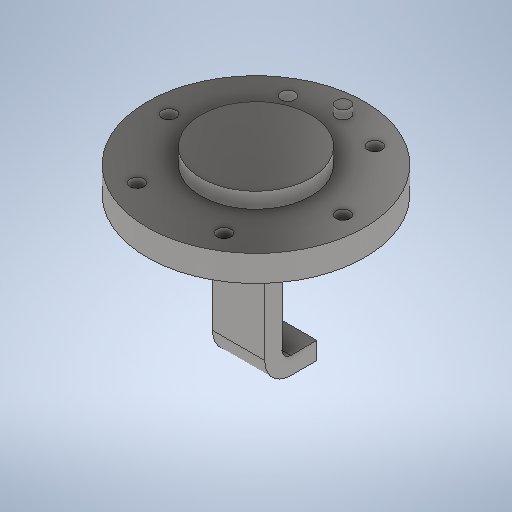
# Autodesk Inventor part: EndEffector
Saved by Autodesk Inventor 2025.1 (Build 291241000, 241)
## iProperties
Created: 2025-01-29
Part Number: EndEffector
Material: Steel, High Strength, Low Alloy
Document SubType Name: Modeling
Designer: yovan
Mass: 2366.38 g
Surface Area: 474.303 cm^2
Volume: 301.45 cm^3
Density: 7.85 g/cm^3
Appearance: Steel - Polished
Author: yovan
Autodesk Inventor part; units mm, degrees
ref_plane "YZ Plane" through (0, 0, 0) normal (1, 0, 0) x (0, 1, 0)
ref_plane "XZ Plane" through (0, 0, 0) normal (0, 1, 0) x (-1, 0, 0)
ref_plane "XY Plane" through (0, 0, 0) normal (0, 0, 1) x (1, 0, 0)
sketch "Sketch3" plane through (0, 0, 0) normal (0, 1, 0) x (-1, 0, 0)
  circle A0 centre (0, 0) radius 62.5
  dimension "d10" = 125
  constraints: 1 centre point, 1 coincident
  measures "d10" diameter of A0
extrude "Extrusion3" add sketch "Sketch3" along normal blind 15
sketch "Sketch9" plane through (0, 0, 0) normal (0, -1, 0) x (1, 0, 0)
  circle A0 centre (0, 0) radius 50
  circle A1 centre (-50, 0) radius 4
  circle A2 centre (-25, -43.3013) radius 4
  circle A3 centre (25, -43.3013) radius 4
  circle A4 centre (50, 0) radius 4
  circle A5 centre (25, 43.3013) radius 4
  circle A6 centre (-25, 43.3013) radius 4
  dimension "d45" = 100
  dimension "d46" = 8
  dimension "d49" = 360
  constraints: 6 centre point, 1 horizontal alignment, 15 other
  measures "d46" diameter of A1
extrude "Extrusion8" cut sketch "Sketch9" against normal blind 20 contours A0 A4 | A0 A4 | A5 A0 | A0 A5 | A3 A0 | A0 A3 | A6 A0 | A0 A6 | A2 A0 | A0 A2 | A1 A0 | A0 A1
sketch "Sketch10" plane through (0, 15, 0) normal (0, 1, 0) x (1, 0, 0)
  circle A0 centre (25, 43.3013) radius 4 projected
  circle A1 centre (0, 0) radius 50
  circle A2 centre (0, 50) radius 4
  circle A3 centre (0, 0) radius 31.5
  dimension "d53" = 8
  dimension "d54" = 63
  constraints: 3 centre point, 2 coincident, 2 point on circle
  measures "d53" diameter of A2
  measures "d54" diameter of A3
extrude "Extrusion9" add sketch "Sketch10" along normal blind 9 contours A3
extrude "Extrusion10" add sketch "Sketch10" along normal blind 5 contours A2 A1 | A1 A2
ref_plane "Work Plane1" through (-20, 0, -20) normal (-1, 0, 0) x (0, 0, 1)
sketch "Sketch14" plane through (-20, 0, -20) normal (-1, 0, 0) x (0, 0, 1)
  line L0 (20, -5) -> (20, -70)
  arc A0 (20, -5) -> (15, 0) centre (15, -5) ccw
  line L1 (15, -75) -> (0, -75)
  arc A1 (15, -75) -> (20, -70) centre (15, -70) ccw
  line L2 (0, -85) -> (15, -85)
  arc A2 (15, -85) -> (30, -70) centre (15, -70) ccw
  line L3 (30, -70) -> (30, -5)
  line L4 (30, -5) -> (30, 0)
  line L5 (30, 0) -> (15, 0)
  line L6 (0, -75) -> (0, -85)
  point P0 (20, 0)
  point P1 (20, -75)
  dimension "d92" = 75
  dimension "d93" = 5
  dimension "d94" = 20
  dimension "d95" = 5
  dimension "d96" = 10
  constraints: 14 end point, 6 point on circle, 4 tangent, 3 centre point, 3 point on line, 3 vertical, 1 horizontal, 1 perpendicular, 2 other
  measures "d92" distance of point (20, 0) point (20, -75)
  measures "d93" radius of A0
  measures "d94" distance of point (20, -75) L1.end
  measures "d95" radius of A1
  measures "d96" distance between parallel lines of L0 L3
extrude "Extrusion16" add sketch "Sketch14" against normal blind 35
extrude "Extrusion17" cut sketch "Sketch14" against normal blind 5
body "Solid2"
